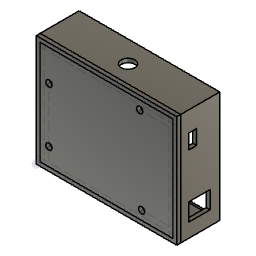
boiteCarteArduinoRIO (Autodesk Fusion 360 design; units mm, degrees)
Autodesk Fusion 360 part; units mm, degrees
sketch "Esquisse1" plane through (0, 0, 0) normal (0, 1, 0) x (1, 0, 0)
  line L0 (0, 0) -> (72, 0)
  line L1 (72, 0) -> (72, -57)
  line L2 (72, -57) -> (0, -57)
  line L3 (0, -57) -> (0, 0)
  line L4 (72, -53) -> (0, -53) construction
  line L5 (72, -4) -> (0, -4) construction
  line L6 (68, -57) -> (68, 0) construction
  line L7 (4, -57) -> (4, 0) construction
  line L8 (68, -50.5) -> (53, -50.5) construction
  circle A0 centre (53, -50.5) radius 1.6
  line L9 (6.5, -4) -> (6.5, -11) construction
  circle A1 centre (6.5, -11) radius 1.6
  line L10 (6.5, -11) -> (6.5, -39) construction
  circle A2 centre (6.5, -39) radius 1.6
  line L11 (68, -6.5) -> (54, -6.5) construction
  circle A3 centre (54, -6.5) radius 1.6
  line L12 (70, -2) -> (70, -55)
  line L13 (70, -55) -> (2, -55)
  line L14 (2, -55) -> (2, -2)
  line L15 (70, -2) -> (2, -2)
  dimension "d1" = 57
  dimension "d2" = 72
  dimension "d3" = 4
  dimension "d4" = 4
  dimension "d5" = 4
  dimension "d6" = 4
  dimension "d7" = 2.5
  dimension "d8" = 15
  dimension "d9" = 3.2
  dimension "d10" = 2.5
  dimension "d11" = 7
  dimension "d12" = 3.2
  dimension "d13" = 35
  dimension "d14" = 3.2
  dimension "d19" = 14
  dimension "d20" = 2.5
  dimension "d21" = 3.2
  dimension "d24" = 2
  dimension "d25" = 2
  dimension "d26" = 2
  dimension "d27" = 2
  constraint horizontal L0
  constraint vertical L1
  constraint horizontal L2
  constraint vertical L3
  constraint coincident L0.start L3.end
  constraint coincident L1 L4.start
  constraint coincident L3 L4.end
  constraint perpendicular L3 L4
  constraint coincident L1 L5.start
  constraint coincident L3 L5.end
  constraint perpendicular L3 L5
  constraint coincident L2 L6.start
  constraint coincident L0 L6.end
  constraint perpendicular L5 L6
  constraint coincident L2 L7.start
  constraint coincident L0 L7.end
  constraint perpendicular L0 L7
  constraint coincident L6 L8.start
  constraint perpendicular L6 L8
  constraint coincident L8.end A0.centre
  constraint coincident L5 L9.start
  constraint perpendicular L5 L9
  constraint coincident L9.end A1.centre
  constraint parallel L9 L10
  constraint coincident L10.end A2.centre
  constraint coincident L6 L11.start
  constraint perpendicular L6 L11
  constraint coincident L11.end A3.centre
  constraint perpendicular L4 L12
  constraint perpendicular L3 L13
  constraint perpendicular L14 L15
  measures "d1" distance of L0.start L2.end
  measures "d2" distance of L1.end L2.end
  measures "d3" distance of L2 L4
  measures "d4" distance of L0 L5
  measures "d5" distance of L3 L7
  measures "d6" distance of L1 L6
  measures "d7" distance of L4 L8
  measures "d8" distance of L6 L8.end
  measures "d9" diameter of A0
  measures "d10" distance of L7 L9
  measures "d11" distance of L5 L9.end
  measures "d12" diameter of A1
  measures "d13" distance of L5 L10.end
  measures "d14" diameter of A2
  measures "d19" distance of L6 L11.end
  measures "d20" distance of L5 L11
  measures "d21" diameter of A3
  measures "d24" distance of L3 L14
  measures "d25" distance of L0 L15
  measures "d26" distance of L1 L12
  measures "d27" distance of L2 L13
extrude "Extrusion1" add sketch "Esquisse1" along normal blind 2 contours L0 L1 L2 L3 | L12 L13 L14 L15 makes body 1
copy_body "Corps->Comp1" bodies 1 removing the originals makes body 2 in component "boiteArduino"
extrude "Extrusion1'" add sketch "Esquisse1" along normal blind 22 separate body contours L0 L1 L2 L3 makes body 3 in component "boiteArduino"
sketch "Esquisse1 (2)" plane through (72, 0, 0) normal (1, 0, 0) x (0, 1, 0) in component "boiteArduino"
  line L0 (0, 57) -> (0, 0)
  line L1 (0, 0) -> (22, 0)
  line L2 (22, 0) -> (22, 57)
  line L3 (22, 57) -> (0, 57)
  line L4 (6.1, 4) -> (9.3822, 4) construction
  line L5 (6.1, 4) -> (6.1, 7.18) construction
  line L6 (0, 0) -> (0, 57) construction
  line L7 (6.1, 7.18) -> (6.1, 16.18)
  line L8 (6.1, 16.18) -> (17.1, 16.18)
  line L9 (17.1, 16.18) -> (17.1, 7.18)
  line L10 (17.1, 7.18) -> (6.1, 7.18)
  dimension "d34" = 4
  dimension "d35" = 3.18
  dimension "d36" = 6.1
  dimension "d41" = 9
  dimension "d42" = 11
  constraint perpendicular L2 L4
  constraint perpendicular L4 L5
  constraint parallel L5 L7
  constraint perpendicular L7 L8
  constraint perpendicular L8 L9
  constraint perpendicular L5 L10
  measures "d34" distance of L1 L4.start
  measures "d35" distance of L4.start L5.end
  measures "d36" distance of L5 L6
  measures "d41" distance of L5.end L7.end
  measures "d42" distance of L5.end L9.end
extrude "Extrusion2" cut sketch "Esquisse1 (2)" against normal blind 9 contours L7 L8 L9 L10 bodies 3 in component "boiteArduino"
sketch "Esquisse2" plane through (72, 0, 0) normal (1, 0, 0) x (0, 1, 0) in component "boiteArduino"
  line L0 (6.1, 16.18) -> (17.1, 16.18)
  line L1 (17.1, 16.18) -> (17.1, 7.18)
  line L2 (17.1, 7.18) -> (6.1, 7.18)
  line L3 (6.1, 7.18) -> (6.1, 16.18)
  line L4 (0, 57) -> (0, 0)
  line L5 (0, 0) -> (22, 0)
  line L6 (22, 0) -> (22, 57)
  line L7 (22, 57) -> (0, 57)
  line L8 (6.1, 16.18) -> (6.1, 39.18) construction
  line L9 (6.1, 39.18) -> (10.1, 39.18)
  line L10 (10.1, 39.18) -> (10.1, 46.68)
  line L11 (10.1, 46.68) -> (6.1, 46.68)
  line L12 (6.1, 46.68) -> (6.1, 39.18)
  dimension "d45" = 23
  dimension "d49" = 7.5
  dimension "d50" = 4
  constraint coincident L0.start L3.end
  constraint perpendicular L0 L8
  constraint horizontal L9
  constraint vertical L10
  constraint horizontal L11
  constraint vertical L12
  measures "d45" distance of L0.start L8.end
  measures "d49" distance of L8.end L11.end
  measures "d50" distance of L10.end L11.end
extrude "Extrusion3" cut sketch "Esquisse2" against normal blind 7 contours L9 L10 L11 L12 bodies 3 in component "boiteArduino"
sketch "Esquisse3" plane through (0, 0, 0) normal (0, 0, -1) x (1, 0, 0) in component "boiteArduino"
  line L0 (72, 0) -> (0, 0)
  line L1 (0, 0) -> (0, -22)
  line L2 (0, -22) -> (72, -22)
  line L3 (72, -22) -> (72, 0)
  line L4 (0, -11) -> (72, -11) construction
  line L5 (36, -22) -> (36, 0) construction
  circle A0 centre (36, -11) radius 3.5
  dimension "d53" = 11
  dimension "d54" = 36
  dimension "d55" = 7
  constraint coincident L1 L4.start
  constraint coincident L3 L4.end
  constraint perpendicular L3 L4
  constraint coincident L2 L5.start
  constraint coincident L0 L5.end
  constraint perpendicular L0 L5
  constraint midpoint L5 A0.centre
  measures "d53" distance of L2 L4
  measures "d54" distance of L3 L5
  measures "d55" diameter of A0
extrude "Extrusion4" cut sketch "Esquisse3" against normal blind 65 contours A0 bodies 3 in component "boiteArduino"
sketch "Esquisse4" plane through (0, 22, 0) normal (0, 1, 0) x (-1, 0, 0) in component "boiteArduino"
  line L0 (-70, 2) -> (-70, 55)
  line L1 (-70, 55) -> (-2, 55)
  line L2 (-2, 55) -> (-2, 2)
  line L3 (-2, 2) -> (-70, 2)
  line L4 (0, 57) -> (-72, 57)
  line L5 (-72, 57) -> (-72, 0)
  line L6 (-72, 0) -> (0, 0)
  line L7 (0, 0) -> (0, 57)
  line L8 (-71, 56) -> (-1, 56)
  line L9 (-1, 56) -> (-1, 1)
  line L10 (-1, 1) -> (-71, 1)
  line L11 (-71, 1) -> (-71, 56)
  line L12 (-72, 57) -> (0, 57)
  dimension "d64" = 1
  dimension "d65" = 1
  constraint horizontal L8
  constraint vertical L9
  constraint horizontal L10
  constraint vertical L11
  measures "d64" distance of L5 L8.start
  measures "d65" distance of L8 L12
extrude "Extrusion5" cut sketch "Esquisse4" against normal blind 2 contours L8 L9 L10 L11 bodies 3 in component "boiteArduino"
component "boiteArduino" placed x (1, 0, 0) y (0, 1, 0) z (0, 0, 1) at (0, 0, 0)
equation "d1 = hauteurMAXoff"
equation "d2 = largeurMAXoff"
equation "d3 = offset"
equation "d4 = offset"
equation "d5 = offset"
equation "d6 = offset"
equation "d7 = distanceCoteCarteTrouVisse"
equation "d8 = distanceTrouVise1"
equation "d9 = rayonCercle"
equation "d10 = distanceCoteCarteTrouVisse"
equation "d11 = distanceTrouVise3"
equation "d12 = rayonCercle"
equation "d13 = distanceTrouVise4"
equation "d14 = rayonCercle"
equation "rayonCercle = 3.2 mm"
equation "offset = 4 mm"
equation "largeurMAXoff = 72 mm"
equation "hauteurMAXoff = 57 mm"
equation "d19 = distanceTrouVise2"
equation "d20 = distanceCoteCarteTrouVisse"
equation "d21 = rayonCercle"
equation "d22 = hauteurbase"
equation "d24 = offset / 2"
equation "d25 = offset / 2"
equation "d26 = offset / 2"
equation "d27 = offset / 2"
equation "hauteurBoite = 20 mm"
equation "hauteurbase = 2 mm"
equation "d32 = hauteurBoite + hauteurbase"
equation "d34 = offset"
equation "d36 = hauteurbase + hauteurSoudure + hauteurCarte"
equation "hauteurCarte = 1.65 mm"
equation "hauteurSoudure = 2.45 mm"
equation "largeurAlimentation = 9 mm"
equation "hauteurAlimentation = 11 mm"
equation "d41 = largeurAlimentation"
equation "d42 = hauteurAlimentation"
equation "d45 = largeurUSBalimentation"
equation "largeurUSBalimentation = 23 mm"
equation "largeurUSB = 7.5 mm"
equation "hauteurUSB = 4 mm"
equation "d49 = largeurUSB"
equation "d50 = hauteurUSB"
equation "d53 = ( hauteurbase + hauteurBoite ) / 2"
equation "d54 = largeurMAXoff / 2"
equation "d55 = cercleCable"
equation "cercleCable = 7 mm"
equation "distanceCoteCarteTrouVisse = 2.5 mm"
equation "distanceTrouVise1 = 15 mm"
equation "distanceTrouVise2 = 14 mm"
equation "distanceTrouVise3 = 7 mm"
equation "distanceTrouVise4 = 35 mm"
equation "d64 = offset / 2 / 2"
equation "d65 = offset / 2 / 2"
equation "hauteurPlexi = 2 mm"
equation "d67 = -hauteurPlexi"
